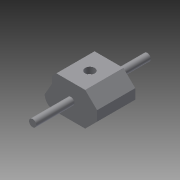
# Autodesk Inventor part: center piece
Saved by Autodesk Inventor 2014 (Build 180170000, 170)
## iProperties
Created: 2017-01-04
Part Number: center piece
Material: Generic
Document SubType Name: Modeling
Designer: lloi
Density: 1 g/cm^3
Appearance: Default
Author: lloi
Autodesk Inventor part; units mm, degrees
ref_plane "YZ Plane" through (0, 0, 0) normal (1, 0, 0) x (0, 1, 0)
ref_plane "XZ Plane" through (0, 0, 0) normal (0, 1, 0) x (-1, 0, 0)
ref_plane "XY Plane" through (0, 0, 0) normal (0, 0, 1) x (1, 0, 0)
sketch "Sketch1" plane through (0, 0, 0) normal (0, 0, 1) x (1, 0, 0)
  line L0 (-77.055, 89.1324) -> (76.1519, 89.1324)
  line L1 (139.6519, 27.5351) -> (139.6519, -25.4)
  line L2 (76.2, -88.852) -> (-88.4125, -88.852)
  line L3 (-139.7639, 88.9233) -> (139.6519, -88.852) construction
  line L4 (139.6519, 89.1324) -> (-139.2125, -88.852) construction
  line L5 (139.6519, 0.1402) -> (139.6519, 27.5351)
  line L6 (139.6519, 0.1402) -> (139.6519, -25.4)
  line L7 (139.6519, 0.1402) -> (139.6519, -25.4)
  line L8 (139.6519, -25.4) -> (76.2, -88.852)
  line L9 (139.6519, 27.5351) -> (76.1519, 89.1324)
  arc A0 (-139.0653, -41.9162) -> (-88.4125, -88.852) centre (-88.4125, -38.052) ccw
  line L10 (-137.5184, -35.1177) -> (-101.1125, 27.9391)
  line L11 (-139.2125, -38.052) -> (-66.4007, -38.052) construction
  line L12 (-101.1125, 27.9391) -> (-101.1125, 65.0749)
  arc A1 (-137.5184, -35.1177) -> (-139.0653, -41.9162) centre (-127.298, -41.0185) ccw
  line L13 (-77.055, 89.1324) -> (-101.1125, 65.0749)
  line L14 (-77.055, 89.1324) -> (-42.3901, 89.1324) construction
  point P0 (0, 0)
  dimension "d9" = 50.8
  constraints: 30 end point, 5 point on circle, 5 point on line, 3 horizontal, 3 tangent, 2 centre point, 1 equal length, 1 parallel, 1 perpendicular
  measures "d9" radius of A0
extrude "Extrusion1" add sketch "Sketch1" along normal mid plane 203.2
sketch "Sketch2" plane through (-77.055, 89.1324, 101.6) normal (0, 1, 0) x (1, 0, 0)
  circle A0 centre (77.055, 101.6) radius 25.4
  dimension "d16" = 50.8
  constraints: 1 centre point, 1 coincident
  measures "d16" diameter of A0
extrude "Extrusion2" cut sketch "Sketch2" against normal blind 38.1
sketch "Sketch4" plane through (0, 0, 101.6) normal (0, 0, 1) x (1, 0, 0)
  circle A0 centre (0, 0) radius 19.05
  dimension "d22" = 38.1
  constraints: 1 centre point, 1 coincident
  measures "d22" diameter of A0
sketch "Sketch5" plane through (0, 0, -101.6) normal (0, 0, -1) x (-1, 0, 0)
  circle A0 centre (0, 0) radius 19.05
  dimension "d23" = 38.1
  constraints: 1 centre point, 1 coincident
  measures "d23" diameter of A0
extrude "Extrusion4" add sketch "Sketch5" along normal blind 203.2
extrude "Extrusion5" add sketch "Sketch4" along normal blind 203.2
sketch "Sketch6" plane through (-101.1125, 27.9391, 101.6) normal (-1, 0, 0) x (0, 0, 1)
  line L0 (-127, 12.4705) -> (-75.6804, 12.4705)
  line L1 (-127, 12.4705) -> (-76.2, 12.4705)
  line L2 (-76.2, 12.4705) -> (-76.2, -116.9301)
  line L3 (-76.2, -116.9301) -> (-127, -116.9301)
  line L4 (-127, -116.9301) -> (-127, 12.4705)
  point P0 (-101.6, -27.9391)
  constraints: 10 end point, 2 parallel, 1 horizontal, 1 perpendicular
extrude "Extrusion6" cut sketch "Sketch6" along normal blind 38.1 and the other way blind 19.05
sketch "Sketch7" plane through (-101.1125, 27.9391, -25.4) normal (0, 0, 1) x (1, 0, 0)
  circle A0 centre (-3.8712, -78.6483) radius 12.7
  point P0 (101.1125, -27.9391)
  dimension "d34" = 25.4
  constraints: 1 centre point
  measures "d34" diameter of A0
extrude "Extrusion7" add sketch "Sketch7" along normal blind 50.8
sketch "Sketch8" plane through (-101.1125, 27.9391, -25.4) normal (0, 0, 1) x (1, 0, 0)
  line L0 (19.05, -116.7911) -> (19.05, 12.4705) projected
  arc A0 (19.05, -116.7911) -> (19.05, 12.4705) centre (-100.0567, -52.1603) ccw
  point P0 (101.1125, -27.9391)
  constraints: 2 point on circle, 1 centre point
extrude "Extrusion8" cut sketch "Sketch8" along normal blind 50.8
sketch "Sketch10" plane through (0, 51.0324, 0) normal (0, 1, 0) x (1, 0, 0)
  circle A0 centre (0, 0) radius 25.4 projected
  circle A1 centre (0, 0) radius 31.75
  dimension "d42" = 63.5
  constraints: 1 centre point, 1 coincident
  measures "d42" diameter of A1
extrude "Extrusion10" cut sketch "Sketch10" along normal blind 5.08
body "Solid1"
